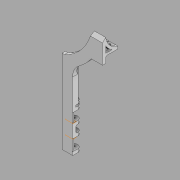
# Autodesk Inventor part: bottom_frame
Saved by Autodesk Inventor 2020 (Build 240168000, 168)
## iProperties
Created: 2020-08-13
Part Number: bottom_frame
Material: Generic
Document SubType Name: Modeling
Designer: alons
Density: 1 g/cm^3
Appearance: Default
Author: alons
Autodesk Inventor part; units mm, degrees
ref_plane "YZ Plane" through (0, 0, 0) normal (1, 0, 0) x (0, 1, 0)
ref_plane "XZ Plane" through (0, 0, 0) normal (0, 1, 0) x (-1, 0, 0)
ref_plane "XY Plane" through (0, 0, 0) normal (0, 0, 1) x (1, 0, 0)
sketch "Sketch2" plane through (0, 0, 0) normal (0, 0, 1) x (1, 0, 0)
  line L0 (0, 12.8113) -> (0, -12.1887)
  line L1 (0, -12.1887) -> (2.5, -12.1887)
  line L2 (2.5, -12.1887) -> (2.5, 12.8113)
  line L3 (2.5, 12.8113) -> (0, 12.8113)
  line L4 (10.05, 37.957) -> (10.05, -69.2724)
  circle A0 centre (10.05, 9.8613) radius 0.5
  circle A1 centre (10.05, -4.8887) radius 0.5
  circle A2 centre (10.05, 1.4113) radius 0.25
  line L5 (2.5, -4.5062) -> (0, -4.5062)
  line L6 (8.3, 22.8113) -> (11.8, 22.8113)
  line L7 (11.8, 22.8113) -> (11.8, 15.8113)
  line L8 (11.8, 15.8113) -> (8.3, 15.8113)
  line L9 (8.3, 15.8113) -> (8.3, 22.8113)
  arc A3 (0, 12.8113) -> (8.3, 22.8113) centre (-6.253, 26.4458) ccw
  arc A4 (2.5, 10.6893) -> (8.3, 15.8113) centre (-6.253, 26.4458) ccw
  point P0 (0, 0)
  point P1 (2.5, -8.7234)
  point P2 (2.5, -1.6342)
  point P3 (10.05, 3.1613)
  dimension "d1" = 25
  dimension "d2" = 2.5
  dimension "d3" = 7.55
  dimension "d4" = 1
  dimension "d15" = 3.5
  dimension "d16" = 7
  dimension "d17" = 3
  dimension "d18" = 15
  constraints: 20 end point, 9 point on line, 5 centre point, 5 perpendicular, 4 point on circle, 2 parallel, 2 vertical, 1 horizontal
  measures "d1" distance of L0.start L0.end
  measures "d2" distance of L0.end L1.end
  measures "d3" distance between parallel lines of L4 L2
  measures "d4" diameter of A0
  measures "d15" distance of L6.start L6.end
  measures "d16" distance of L6.end L7.end
  measures "d17" distance between parallel lines of L8 L3
  measures "d18" radius of A3
extrude "Extrusion1" add sketch "Sketch2" along normal blind 1 contours L3 L2 L5 L0 | A3 L9 A4 L2 L3 | L5 L2 L1 L0 | L6 L4 L8 L9 | L6 L7 L8 L4
sketch "Sketch3" plane through (0, 0, 0) normal (0, 0, -1) x (-1, 0, 0)
  line L0 (-0.75, 0.6623) -> (-1.75, 0.6623)
  line L1 (-1.75, 0.6623) -> (-1.75, 11.6623)
  line L2 (-1.75, 11.6623) -> (-0.75, 11.6623)
  line L3 (-0.75, 11.6623) -> (-0.75, 0.6623)
  line L4 (-2.5, -12.1887) -> (-2.5, 10.6893) projected
  line L5 (0, 12.8113) -> (0, -12.1887) projected
  line L6 (-2.5, -0.0877) -> (0, -0.0877)
  line L7 (0, -0.0877) -> (0, 12.4123)
  line L8 (0, 12.4123) -> (-2.5, 12.4123)
  line L9 (-2.5, 12.4123) -> (-2.5, -0.0877)
  line L10 (-1.75, 0.6623) -> (-2.5, 0.6623)
  line L11 (-0.75, 0.6623) -> (0, 0.6623)
  line L12 (-1.75, 11.6623) -> (-2.5, 11.6623)
  line L13 (-0.75, 11.6623) -> (0, 11.6623)
  point P0 (0, 0)
  point P1 (-10.05, 1.4113)
  point P2 (-2.5, -1.6342)
  dimension "d21" = 0.75
  dimension "d22" = 0.75
  dimension "d23" = 10.251
  dimension "d24" = 0.75
  dimension "d27" = 11
  constraints: 24 end point, 6 point on line, 4 parallel, 4 perpendicular, 1 horizontal, 3 other
  measures "d21" distance between parallel lines of L4 L1
  measures "d22" distance between parallel lines of L5 L3
  measures "d23" distance from line of point (-10.05, 1.411) L2
  measures "d24" distance between parallel lines of L0 L6
  measures "d27" distance of L2.end L0.start
extrude "Extrusion6" add sketch "Sketch3" along normal blind 0.75 contours L11 L5 L6 L4 L10 L0 | L3 L13 L5 L11 | L10 L4 L9 L12 L1 | L2 L12 L9 L8 L5 L13
sketch "Sketch7" plane through (0.75, 0.6623, 0) normal (0, 1, 0) x (1, 0, 0)
  line L0 (1, 0) -> (0, 0) projected
  line L1 (1, 0) -> (1, 0.75) projected
  line L2 (0, 0.75) -> (1, 0.75) projected
  line L3 (0, 0) -> (0, 0.75) projected
  line L4 (1.75, 0.75) -> (-0.75, 0.75) projected
  line L5 (0.5, 0.75) -> (0.5, 0)
  line L6 (-0.75, 0) -> (1.75, 0) projected
  circle A0 centre (0.5, 0.75) radius 0.75
  point P0 (1, 0.191)
  point P1 (1.25, 0.75)
  point P2 (-0.25, 0.75)
  point P3 (0, 0.191)
  constraints: 2 end point, 2 midpoint, 1 coincident, 3 other
extrude "Extrusion7" cut sketch "Sketch7" along normal up to surface (11 mm away) contours L1 L4 A0 | A0 L4 L3
extrude "Extrusion8" add sketch "Sketch7" along normal up to surface (11 mm away) contours L0 A0 L1 | L0 L3 A0
sketch "Sketch8" plane through (0, 0, -0.75) normal (0, 0, -1) x (-1, 0, 0)
  line L0 (-2, 11.6623) -> (-0.5, 11.6623) projected
  line L1 (-0.5, 11.6623) -> (-0.5, 0.6623) projected
  line L2 (-0.5, 0.6623) -> (-2, 0.6623) projected
  line L3 (-2, 0.6623) -> (-2, 11.6623) projected
  line L4 (0, -0.0877) -> (0, 12.4123) projected
  line L5 (0, 12.4123) -> (-2.5, 12.4123) projected
  line L6 (-2.5, 12.4123) -> (-2.5, -0.0877) projected
  line L7 (-2.5, -0.0877) -> (0, -0.0877) projected
  line L8 (-0.5, 0.6623) -> (0, 0.6623)
  line L9 (0, 12.8113) -> (0, -12.1887) projected
  line L10 (-0.5, 0.6623) -> (-2, 0.6623) projected
  line L11 (-2, 0.6623) -> (-2.5, 0.6623)
  line L12 (-2, 11.6623) -> (-0.5, 11.6623) projected
  line L13 (-0.5, 11.6623) -> (0, 11.6623)
  line L14 (-2, 11.6623) -> (-2.5, 11.6623)
  point P0 (0, 0)
  constraints: 8 end point, 6 point on line, 2 perpendicular
extrude "Extrusion9" add sketch "Sketch8" along normal blind 1 contours L14 L6 L5 L4 L13 L0 | L2 L8 L4 L7 L6 L11
sketch "Sketch9" plane through (0, 12.4123, 0) normal (0, 1, 0) x (1, 0, 0)
  circle A0 centre (1.25, 0.75) radius 0.75 projected
  line L0 (2.5, 0.75) -> (0, 0.75) projected
  line L1 (1.25, 0.75) -> (1.25, 1.75)
  line L2 (0, 1.75) -> (2.5, 1.75) projected
  line L3 (2.5, 0.75) -> (2.5, 1.75) projected
  line L4 (0, 0.75) -> (0.5, 0.75) projected
  arc A1 (2.5, 0.75) -> (0, 0.75) centre (1.25, 0.4688) ccw
  line L5 (0, 0) -> (0, 1.75) projected
  circle A2 centre (1.25, 0.75) radius 0.25
  dimension "d44" = 0.5
  constraints: 3 point on circle, 2 centre point, 2 end point, 1 coincident, 1 horizontal alignment, 1 midpoint
  measures "d44" diameter of A2
extrude "Extrusion10" cut sketch "Sketch9" against normal through all contours L5 L2 A1 | A2 L1 L0 | L0 A2 | A1 L2 L3 | L0 L1 A2
sketch "Sketch11" plane through (0, 0, 0) normal (0, 0, -1) x (-1, 0, 0)
  arc A0 (-8.3, 22.8113) -> (0, 12.8113) centre (6.253, 26.4458) ccw projected
  line L0 (-11.8, 22.8113) -> (-8.3, 22.8113) projected
  line L1 (-11.8, 15.8113) -> (-11.8, 22.8113) projected
  line L2 (-8.3, 15.8113) -> (-11.8, 15.8113) projected
  arc A1 (-8.3, 15.8113) -> (-2.5, 10.6893) centre (6.253, 26.4458) ccw projected
  line L3 (-2.5, -12.1887) -> (-2.5, -0.0877) projected
  line L4 (-8.3, 15.8113) -> (-8.3, 22.8113)
  line L5 (-8.3, 17.8113) -> (-11.8, 17.8113)
  line L6 (-8.3, 18.5613) -> (-11.8, 18.5613)
  line L7 (0, -12.1887) -> (-2.5, -12.1887) projected
  line L8 (0, -0.0877) -> (-2.5, -0.0877) projected
  line L9 (-2.5, 10.6893) -> (-2.5, 12.4123) projected
  line L10 (-2.5, 12.4123) -> (0, 12.4123) projected
  line L11 (0, -0.0877) -> (0, -12.1887) projected
  line L12 (0, 12.8113) -> (0, 12.4123) projected
  point P0 (0, 0)
  dimension "d50" = 2
  dimension "d51" = 0.75
  constraints: 6 end point, 4 point on line, 2 perpendicular, 1 vertical
  measures "d50" distance between parallel lines of L5 L2
  measures "d51" distance between parallel lines of L6 L5
extrude "Extrusion12" add sketch "Sketch11" along normal blind 3.8 contours L4 L5 L1 L6
sketch "Sketch12" plane through (8.3, 18.5613, 0) normal (0, 1, 0) x (1, 0, 0)
  line L0 (3.5, 0) -> (0, 0) projected
  line L1 (3.5, 0) -> (3.5, 3.8) projected
  line L2 (0, 3.8) -> (3.5, 3.8) projected
  line L3 (0, 0) -> (0, 3.8) projected
  line L4 (0, 3.8) -> (3.5, 3.8) projected
  line L5 (1.75, 3.8) -> (1.75, 0)
  line L6 (3.5, 0) -> (0, 0) projected
  circle A0 centre (1.75, 3) radius 0.25
  line L7 (1.75, 3.25) -> (3.4773, 3.25)
  line L8 (3.5, 0) -> (3.5, 3.8) projected
  line L9 (1.75, 3.25) -> (0, 3.25)
  line L10 (0, 0) -> (0, 3.8) projected
  point P0 (-8.3, 0)
  dimension "d54" = 0.5
  dimension "d55" = 3.25
  constraints: 6 end point, 3 point on line, 2 midpoint, 2 perpendicular, 1 vertical alignment, 2 other
  measures "d55" distance between parallel lines of L0 L7
extrude "Extrusion13" cut sketch "Sketch12" against normal through all contours A0 L5 | L5 A0
fillet "Fillet7" radius 5 1 edges at (2.5, 10.6893, 0.5)
sketch "Sketch14" plane through (0, -12.1887, 0) normal (0, -1, 0) x (1, 0, 0)
  line L0 (2.5, 0) -> (0.25, 0) projected
  line L1 (2.5, 1) -> (2.5, 0) projected
  line L2 (0, 1) -> (2.5, 1) projected
  line L3 (0, 0) -> (0, 1) projected
  line L4 (0, 0) -> (2.5, 0) projected
extrude "Extrusion15" add sketch "Sketch14" along normal blind 1
ref_plane "Work Plane1" through (0, -8.7237, 0) normal (0, 1, 0) x (1, 0, 0)
sketch "Sketch17" plane through (11.8, 15.8113, 1) normal (1, 0, 0) x (0, 0, -1)
  line L0 (1, 0) -> (1, 2) projected
  line L1 (1, 2) -> (4.8, 2) projected
  line L2 (4.8, 2.75) -> (4.8, 2) projected
  line L3 (1, 2.75) -> (4.8, 2.75) projected
  line L4 (1, 2.75) -> (1, 7) projected
  line L5 (1, 7) -> (0, 7) projected
  line L6 (0, 0) -> (0, 7) projected
  line L7 (1, 0) -> (0, 0) projected
  arc A0 (1, 7) -> (4.8, 2.75) centre (5.9623, 7.613) ccw
  arc A1 (1, 4.7437) -> (2.9278, 2.75) centre (5.9623, 7.613) ccw
  point P0 (1, -15.8113)
  dimension "d89" = 5
  constraints: 4 point on circle, 2 centre point, 2 point on line
  measures "d89" radius of A0
extrude "Extrusion18" add sketch "Sketch17" against normal blind 0.75 contours L3 A1 L4 A0
ref_plane "Work Plane2" through (8.3, 15.8113, 1) normal (1, 0, 0) x (0, 0, -1)
sketch "Sketch18" plane through (8.3, 15.8113, 1) normal (1, 0, 0) x (0, 0, -1)
  arc A0 (1, 7) -> (4.8, 2.75) centre (5.9623, 7.613) ccw projected
  arc A1 (1, 4.7437) -> (2.9278, 2.75) centre (5.9623, 7.613) ccw projected
  line L0 (1, 2.75) -> (1, 2) projected
  line L1 (1, 2.75) -> (4.8, 2.75) projected
  line L2 (4.8, 2) -> (4.8, 2.75) projected
  line L3 (1, 2) -> (4.8, 2) projected
  line L4 (1, -3) -> (1, 7) projected
  point P0 (1, -15.8113)
  point P1 (2.9278, 2.75)
extrude "Extrusion19" add sketch "Sketch18" along normal blind 0.75 contours A0 L1 A1 L4
chamfer "Chamfer4" distance 1 angle 45 1 edges at (10.05, 22.8113, 1)
sketch "Sketch19" plane through (8.3, 17.8113, 0) normal (0, -1, 0) x (1, 0, 0)
  circle A0 centre (1.75, -3) radius 0.25 projected
  line L0 (0, 0) -> (3.5, 0) projected
  line L1 (0, 0) -> (0, -3.8) projected
  line L2 (3.5, -3.8) -> (0, -3.8) projected
  line L3 (3.5, 0) -> (3.5, -3.8) projected
  circle A1 centre (1.75, -3) radius 0.25 projected
  line L4 (1.75, -3) -> (1.75, 0)
  line L5 (2.75, 0) -> (0.75, 0) projected
  line L6 (1.75, -3) -> (0, -3)
  line L7 (0, 0) -> (0, -3.8) projected
  line L8 (1.75, -3) -> (3.5, -3)
  line L9 (3.5, 0) -> (3.5, -3.8) projected
  line L10 (2.75, 0) -> (2.75, -1.9278) projected
  line L11 (2.75, -1.9278) -> (2.75, -3.8) projected
  line L12 (0.75, -3.8) -> (0.75, -1.9278) projected
  line L13 (0.75, -1.9278) -> (0.75, 0) projected
  line L14 (1.75, -2.2) -> (0, -2.2)
  line L15 (1.75, -2.2) -> (3.5, -2.2)
  point P0 (-8.3, 0)
  point P1 (2.75, -2.2)
  point P2 (0.75, -2.2)
  dimension "d98" = 0.8
  dimension "d99" = 0.8
  constraints: 10 end point, 3 point on line, 2 parallel, 1 midpoint, 1 perpendicular
  measures "d98" distance between parallel lines of L6 L14
  measures "d99" distance between parallel lines of L8 L15
extrude "Extrusion20" cut sketch "Sketch19" against normal through all contours L14 L12 L13 L0 L4 | L4 L0 L10 L11 L15
chamfer "Chamfer5" distance 0.25 angle 45 1 edges at (10.05, 17.8113, -3.8)
fillet "Fillet13" radius 0.5 2 edges at (11.425, 17.8113, 0) (8.675, 17.8113, 0)
sketch "Sketch20" plane through (0, 12.8113, 0) normal (-1, 0, 0) x (0, 0, 1)
  line L0 (-0.75, -0.399) -> (-0.75, -1.149) projected
  line L1 (-0.75, -12.149) -> (-0.75, -1.149) projected
  line L2 (-0.75, -12.149) -> (-0.75, -12.899) projected
  line L3 (0, -12.899) -> (-0.75, -12.899) projected
  line L4 (0, -12.899) -> (0, -26) projected
  line L5 (1, -26) -> (0, -26) projected
  line L6 (1, 0) -> (1, -26) projected
  line L7 (0, 0) -> (1, 0) projected
  line L8 (0, 0) -> (0, -0.399) projected
  line L9 (0, -0.399) -> (-0.75, -0.399) projected
  line L10 (0, -12.899) -> (-0.75, -12.899) projected
  line L11 (0, -12.899) -> (0, -0.399)
  point P0 (0, -12.8113)
  constraints: 2 end point, 1 perpendicular
extrude "Extrusion21" add sketch "Sketch20" along normal blind 0.75 contours L8 L7 L6 L5 L4 L11
sketch "Sketch21" plane through (0, -13.1887, 0) normal (0, -1, 0) x (1, 0, 0)
  circle A0 centre (1.25, -0.75) radius 0.25 projected
  circle A1 centre (1.25, -0.75) radius 1
  line L0 (2.5, 0) -> (2.5, 1) projected
  line L1 (2.5, 1) -> (1.9114, 0)
  line L2 (2.5, 1) -> (-0.75, 1) projected
  arc A2 (0, -0.75) -> (2.5, -0.75) centre (1.25, -0.4688) ccw projected
  circle A3 centre (1.25, -0.75) radius 0.25 projected
  arc A4 (0, -0.75) -> (2.5, -0.75) centre (1.25, -0.4688) ccw projected
  line L3 (2.5, 0) -> (2.5, -0.75) projected
  line L4 (0, 0) -> (2.5, 0) projected
  line L5 (0, 0) -> (0, -0.75) projected
  point P0 (0, 0)
  point P1 (2.5, -0.75)
  point P2 (0, -0.75)
  dimension "d108" = 2
  dimension "d109" = 59.521
  constraints: 2 end point, 1 coincident, 3 other
  measures "d109" angle of L2 L1
sketch "Sketch22" plane through (0, -8.7237, 0) normal (0, 1, 0) x (1, 0, 0)
  line L0 (2.5, 0) -> (-0.75, 0) projected
  line L1 (2.5, 0) -> (2.5, -1) projected
  circle A0 centre (1.25, 0.75) radius 1 projected
  circle A1 centre (1.25, 0.75) radius 0.25 projected
  line L2 (2.5, -1) -> (1.9114, 0) projected
  point P0 (0, 0)
  point P1 (1.9114, 0)
  point P2 (1.9114, 0)
  point P3 (0.5886, 0)
extrude "Extrusion22" cut sketch "Sketch22" against normal blind 3.465 contours L1 L2 L0 | A0 L0 picked at (1.0955, -0.0454)
ref_plane "Work Plane3" through (0, -4.5067, 0) normal (0, 1, 0) x (1, 0, 0)
sketch "Sketch23" plane through (0, -4.5067, 0) normal (0, 1, 0) x (1, 0, 0)
  line L0 (0.5886, 0) -> (1.9114, 0) projected
  arc A0 (0.5886, 0) -> (1.9114, 0) centre (1.25, 0.75) ccw projected
  line L1 (2.5, -1) -> (1.9114, 0) projected
  line L2 (2.5, 0) -> (2.5, -1) projected
  line L3 (1.9114, 0) -> (2.5, 0) projected
  point P0 (0, 0)
  point P1 (1.9114, 0)
  point P2 (1.9114, 0)
  point P3 (1.9114, 0)
  point P4 (1.9114, 0)
extrude "Extrusion23" cut sketch "Sketch23" along normal blind 2.872
extrude "Extrusion24" add sketch "Sketch21" against normal up to surface (1 mm away) contours A1 L4 | A1 L4 L3 A2 | A2 L5 L4 A1 picked at (1.2399, -0.1673)
sketch "Sketch24" plane through (0, -4.5067, 0) normal (0, 1, 0) x (1, 0, 0)
  circle A0 centre (1.25, 0.75) radius 0.25 projected
  line L0 (2.5, 0.75) -> (2.5, -1) projected
  line L1 (2.5, -1) -> (-0.75, -1) projected
  line L2 (-0.75, 0) -> (-0.75, -1) projected
  line L3 (0, 0) -> (-0.75, 0) projected
  line L4 (0, 0) -> (0, 0.75) projected
  arc A1 (2.5, 0.75) -> (0, 0.75) centre (1.25, 0.4688) ccw projected
  line L5 (1.9114, 0) -> (2.5, 0) projected
  line L6 (0.5886, 0) -> (1.9114, 0) projected
  line L7 (0.5886, 0) -> (0, 0)
  point P0 (0, 0)
  constraints: 2 end point, 1 horizontal
extrude "Extrusion25" add sketch "Sketch24" against normal blind 1 contours L0 L5 L6 L7 L4 A1
sketch "Sketch25" plane through (0, -8.7237, 0) normal (0, 1, 0) x (1, 0, 0)
  line L0 (0, 0) -> (0, 0.75) projected
  arc A0 (2.5, 0.75) -> (0, 0.75) centre (1.25, 0.4688) ccw projected
  line L1 (2.5, 0.75) -> (2.5, 0) projected
  line L2 (0, 0) -> (2.5, 0) projected
  circle A1 centre (1.25, 0.75) radius 0.25 projected
  point P0 (0, 0)
extrude "Extrusion26" add sketch "Sketch25" along normal blind 1
sketch "Sketch26" plane through (0, -1.6347, 0) normal (0, -1, 0) x (1, 0, 0)
  line L0 (0, 0) -> (0, -0.75) projected
  arc A0 (0, -0.75) -> (2.5, -0.75) centre (1.25, -0.4688) ccw projected
  line L1 (2.5, -0.75) -> (2.5, 0) projected
  line L2 (0, 0) -> (2.5, 0) projected
  circle A1 centre (1.25, -0.75) radius 0.25 projected
  point P0 (0, 0)
extrude "Extrusion27" add sketch "Sketch26" against normal blind 1
fillet "Fillet15" radius 0.5 8 edges at (2.5, 10.1962, 0) (1.25, -5.5067, 0) (1.25, -7.7237, 0) (0, -12.6887, 0) (0, -8.2237, 0) (0, -5.0067, 0) (0, -1.1347, 0) (0, 6.1623, 0)
body "Solid1"
